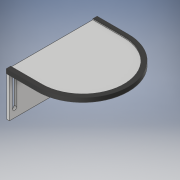
# Autodesk Inventor part: Glas und Flaschenboden
Saved by Autodesk Inventor 2019 (Build 230136000, 136)
## iProperties
Created: 2018-09-20
Part Number: Glas und Flaschenboden
Material: Generisch
Document SubType Name: Modeling
Designer: nico-
Density: 1 g/cm^3
Appearance: Vorgabe
Author: nico-
Autodesk Inventor part; units mm, degrees
ref_plane "YZ Plane" through (0, 0, 0) normal (1, 0, 0) x (0, 1, 0)
ref_plane "XZ Plane" through (0, 0, 0) normal (0, 1, 0) x (-1, 0, 0)
ref_plane "XY Plane" through (0, 0, 0) normal (0, 0, 1) x (1, 0, 0)
sketch "Skizze1" plane through (0, 0, 0) normal (0, 0, 1) x (1, 0, 0)
  line L0 (0, 0) -> (0, -50)
  line L1 (0, 0) -> (50, 0) construction
  line L2 (0, -50) -> (3, -50)
  line L3 (3, -50) -> (3, -3)
  line L4 (3, -3) -> (88, -3)
  line L5 (88, -3) -> (88, 0)
  line L6 (88, 0) -> (0, 0)
  dimension "d0" = 50
  dimension "d1" = 90
  dimension "d2" = 3
  dimension "d3" = 47
  dimension "d4" = 85
  dimension "d5" = 90
  constraints: 14 end point, 6 perpendicular, 1 horizontal, 1 vertical
  measures "d0" distance of L0.start L0.end
  measures "d1" angle of L0 L1
  measures "d2" distance of L0.end L2.end
  measures "d3" distance of L2.end L3.end
  measures "d4" distance of L3.end L4.end
  measures "d5" angle of L3 L4
extrude "Extrusion1" add sketch "Skizze1" along normal mid plane 104
fillet "Rundung1" radius 52 2 edges at (88, -1.5, -52) (88, -1.5, 52)
sketch "Skizze2" plane through (3, -50, 52) normal (1, 0, 0) x (0, 0, -1)
  line L0 (3.5, 40) -> (8.5, 40)
  line L1 (8.5, 40) -> (8.5, 10)
  line L2 (8.5, 10) -> (3.5, 10)
  line L3 (3.5, 10) -> (3.5, 40)
  arc A0 (8.5, 40) -> (3.5, 40) centre (6, 40) ccw
  arc A1 (3.5, 10) -> (8.5, 10) centre (6, 10) ccw
  line L4 (0, 0) -> (0, 47) projected
  point P0 (52, 50)
  dimension "d9" = 5
  dimension "d10" = 30
  dimension "d27" = 6
  constraints: 8 end point, 4 point on circle, 2 centre point, 2 midpoint, 2 parallel, 1 horizontal, 1 perpendicular
  measures "d9" distance of L1.end L2.end
  measures "d10" distance of L0.end L1.end
  measures "d27" distance from line of L4 A1.centre
extrude "Extrusion2" cut sketch "Skizze2" against normal blind 3
sketch "Skizze3" plane through (3, -50, 52) normal (1, 0, 0) x (0, 0, -1)
  line L0 (100.5, 40) -> (95.5, 40)
  line L1 (95.5, 40) -> (95.5, 10)
  line L2 (95.5, 10) -> (100.5, 10)
  line L3 (100.5, 10) -> (100.5, 40)
  arc A0 (100.5, 40) -> (95.5, 40) centre (98, 40) ccw
  arc A1 (95.5, 10) -> (100.5, 10) centre (98, 10) ccw
  line L4 (104, 47) -> (104, 0) projected
  point P0 (52, 50)
  dimension "d13" = 5
  dimension "d14" = 30
  dimension "d28" = 6
  constraints: 8 end point, 4 point on circle, 2 centre point, 2 midpoint, 2 parallel, 1 horizontal, 1 perpendicular
  measures "d13" distance of L2.end L1.end
  measures "d14" distance of L1.end L0.end
  measures "d28" distance from line of L4 A1.centre
extrude "Extrusion3" cut sketch "Skizze3" against normal blind 3
sketch "Skizze4" plane through (0, 0, 52) normal (0, 1, 0) x (1, 0, 0)
  arc A0 (36, -0.5) -> (36, 104.5) centre (36, 52) ccw
  line L0 (36, 52) -> (36, -0.5) construction
  line L1 (36, 52) -> (88.5, 52) construction
  line L2 (36, 52) -> (36, 104.5) construction
  arc A1 (36, 4.5) -> (36, 99.5) centre (36, 52) ccw
  line L3 (36, 52) -> (36, 4.5) construction
  line L4 (36, 52) -> (83.5, 52) construction
  line L5 (36, 99.5) -> (0, 99.5)
  line L6 (0, 95.5) -> (0, 100.5) projected
  line L7 (36, 104) -> (3, 104) projected
  line L8 (36, -0.5) -> (0, -0.5)
  line L9 (0, -0.5) -> (0, 4.5)
  line L10 (36, 4.5) -> (0, 4.5)
  line L11 (0, 99.5) -> (0, 104.5)
  line L12 (0, 104.5) -> (36, 104.5)
  line L13 (0, 0) -> (0, 104) projected
  point P0 (0, 52)
  dimension "d17" = 52.5
  dimension "d18" = 90
  dimension "d19" = 180
  dimension "d20" = 47.5
  dimension "d21" = 90
  constraints: 22 end point, 6 point on line, 4 horizontal, 4 perpendicular, 4 point on circle, 2 centre point, 1 coincident
  measures "d17" radius of A0
  measures "d18" angle of L0 L1
  measures "d19" angle of L0 L2
  measures "d20" radius of A1
  measures "d21" angle of L3 L4
extrude "Extrusion4" add sketch "Skizze4" along normal blind 1 and the other way blind 4 contours L8 L9 L10 A1 L5 L6 L11 L12 A0
